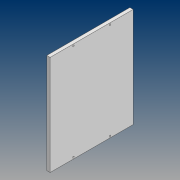
# Autodesk Inventor part: 10_Tam_go_mat_top
Saved by Autodesk Inventor 2021 (Build 250183000, 183)
## iProperties
Created: 2024-04-01
Part Number: 10_Tam_go_mat_top
Material: Generic
Document SubType Name: Modeling
Designer: Admin
Density: 1 g/cm^3
Appearance: Default
Author: Admin
Autodesk Inventor part; units mm, degrees
ref_plane "YZ Plane" through (0, 0, 0) normal (1, 0, 0) x (0, 1, 0)
ref_plane "XZ Plane" through (0, 0, 0) normal (0, 1, 0) x (-1, 0, 0)
ref_plane "XY Plane" through (0, 0, 0) normal (0, 0, 1) x (1, 0, 0)
sketch "Sketch1" plane through (0, 0, 0) normal (1, 0, 0) x (0, 1, 0)
  line L0 (-150, 125) -> (150, 125)
  line L1 (150, 125) -> (150, -125)
  line L2 (150, -125) -> (-150, -125)
  line L3 (-150, -125) -> (-150, 125)
  line L4 (-150, 125) -> (150, -125) construction
  line L5 (150, 125) -> (-150, -125) construction
  point P0 (0, 0)
  dimension "d0" = 250
  dimension "d1" = 300
  constraints: 12 end point, 2 midpoint, 2 parallel, 1 horizontal, 1 perpendicular
  measures "d0" distance of L0.end L1.end
  measures "d1" distance of L1.end L2.end
extrude "Extrusion1" add sketch "Sketch1" along normal blind 10
sketch "Sketch2" plane through (0, 0, 0) normal (-1, 0, 0) x (0, 0, 1)
  line L0 (-125, -150) -> (-125, 150) projected
  line L1 (125, -150) -> (-125, -150) projected
  line L2 (125, 150) -> (125, -150) projected
  line L3 (-125, 150) -> (125, 150) projected
  line L4 (120, -145) -> (-120, -145)
  line L5 (-120, -145) -> (-120, 145)
  line L6 (-120, 145) -> (120, 145)
  line L7 (120, 145) -> (120, -145)
  line L8 (0, -210) -> (0, 210) construction
  line L9 (-175, 0) -> (175, 0) construction
  point P0 (0, 0)
  point P1 (0, 145)
  point P2 (55, 145)
  point P3 (0, -145)
  point P4 (-55, 145)
  dimension "d4" = 5
  dimension "d7" = 70
  dimension "d8" = 70
  constraints: 8 end point, 2 midpoint, 2 point on line, 3 other
  measures "d4" distance between parallel lines of L2 L7
  measures "d7" distance from line of point (-55, 145) L0
  measures "d8" distance from line of L2 point (55, 145)
hole "Hole1" at (0, 145, 55) at (0, 145, -55) direction (1, 0, 0) diameter 5 end through all
mirror "Mirror1" about plane through (0, 0, 0) normal (0, 1, 0) of "Hole1"
body "Solid1"
